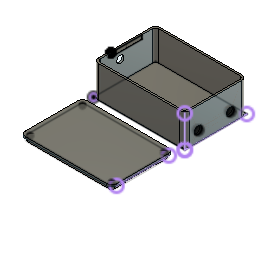
esp12_triac v6 (Autodesk Fusion 360 design; units mm, degrees)
Autodesk Fusion 360 part; units mm, degrees
sketch "Base" plane through (0, 0, 0) normal (0, 1, 0) x (1, 0, 0) in component "Case"
  line L0 (0, 0) -> (75, 0)
  line L1 (75, 0) -> (75, 51)
  line L2 (75, 51) -> (0, 51)
  line L3 (0, 51) -> (0, 0)
  dimension "d6" = 75
  dimension "d7" = 51
  constraint horizontal L0
  constraint vertical L1
  constraint horizontal L2
  constraint vertical L3
  constraint coincident L0.start L3.end
  measures "d6" distance of L0.start L0.end
  measures "d7" distance of L0.start L2.end
extrude "Extrude1" add sketch "Base" along normal blind 26 makes body 1 in component "Case"
fillet "Fillet1" radius 4 4 edges at (75, 13, 0) (0, 13, 0) (75, 13, -51) (0, 13, -51) on bodies 1 in component "Case"
shell "Shell1" thickness 1.5 removed faces 1 at (48.6667, 26, -17) on bodies 1 in component "Case"
sketch "Knob" plane through (1.5, 0, 0) normal (1, 0, 0) x (0, 0, -1) in component "Case"
  line L0 (47, 1.5) -> (47, 26)
  line L1 (47, 26) -> (4, 26)
  line L2 (4, 26) -> (4, 1.5)
  line L3 (4, 1.5) -> (47, 1.5)
  line L4 (12.75, 26) -> (38.25, 26)
  line L5 (38.25, 26) -> (38.25, 23)
  line L6 (38.25, 23) -> (12.75, 23)
  line L7 (12.75, 23) -> (12.75, 26)
  line L8 (25.5, 26) -> (25.5, 23) construction
  dimension "d12" = 25.5
  dimension "d13" = 3
  constraint horizontal L4
  constraint vertical L5
  constraint horizontal L6
  constraint vertical L7
  constraint coincident L1 L4.start
  constraint midpoint L1 L8.start
  constraint midpoint L6 L8.end
  constraint vertical L8
  measures "d12" distance of L5.end L6.end
  measures "d13" distance of L4.end L5.end
extrude "Extrude2" add sketch "Knob" along normal blind 6 draft -45 contours L1 L4 L5 L6 L7 bodies 1 in component "Case"
ref_plane "WorkPlane2" through (37.5, 13, -25.5) normal (-1, 0, 0) x (0, 0, 1) in component "Case"
mirror "Mirror1" about plane through (37.5, 13, -25.5) normal (-1, 0, 0) of "Extrude2" in component "Case"
sketch "Top" plane through (0, 26, 0) normal (0, 1, 0) x (-1, 0, 0) in component "Top Cover"
  line L0 (-75, -4) -> (-75, -47)
  arc A0 (-75, -47) -> (-71, -51) centre (-71, -47) ccw
  line L1 (-71, -51) -> (-4, -51)
  arc A1 (-4, -51) -> (0, -47) centre (-4, -47) ccw
  line L2 (0, -47) -> (0, -4)
  arc A2 (0, -4) -> (-4, 0) centre (-4, -4) ccw
  line L3 (-4, 0) -> (-71, 0)
  arc A3 (-71, 0) -> (-75, -4) centre (-71, -4) ccw
  line L4 (-73.5, -12.75) -> (-73.5, -4)
  arc A4 (-71, -1.5) -> (-73.5, -4) centre (-71, -4) ccw
  line L5 (-71, -1.5) -> (-4, -1.5)
  arc A5 (-1.5, -4) -> (-4, -1.5) centre (-4, -4) ccw
  line L6 (-1.5, -4) -> (-1.5, -12.75)
  line L7 (-1.5, -12.75) -> (-1.5, -38.25)
  line L8 (-1.5, -38.25) -> (-1.5, -47)
  arc A6 (-4, -49.5) -> (-1.5, -47) centre (-4, -47) ccw
  line L9 (-4, -49.5) -> (-71, -49.5)
  arc A7 (-73.5, -47) -> (-71, -49.5) centre (-71, -47) ccw
  line L10 (-73.5, -47) -> (-73.5, -38.25)
  line L11 (-73.5, -38.25) -> (-73.5, -12.75)
extrude "Extrude1'" add sketch "Top" along normal blind 1.5 separate body contours L0 A0 L1 A1 L2 A2 L3 A3 | L4 A4 L5 A5 L6 L7 L8 A6 L9 A7 L10 L11 makes body 2 in component "Top Cover"
sketch "Lip" plane through (0, 26, 0) normal (0, -1, 0) x (1, 0, 0) in component "Top Cover"
  arc A0 (75, -4) -> (71, 0) centre (71, -4) ccw
  line L0 (71, 0) -> (4, 0)
  arc A1 (4, 0) -> (0, -4) centre (4, -4) ccw
  line L1 (0, -4) -> (0, -47)
  arc A2 (0, -47) -> (4, -51) centre (4, -47) ccw
  line L2 (4, -51) -> (71, -51)
  arc A3 (71, -51) -> (75, -47) centre (71, -47) ccw
  line L3 (75, -47) -> (75, -4)
  line L4 (73.3, -47) -> (73.3, -4)
  arc A4 (73.3, -4) -> (71, -1.7) centre (71, -4) ccw
  line L5 (71, -1.7) -> (4, -1.7)
  arc A5 (4, -1.7) -> (1.7, -4) centre (4, -4) ccw
  line L6 (1.7, -4) -> (1.7, -47)
  arc A6 (1.7, -47) -> (4, -49.3) centre (4, -47) ccw
  line L7 (4, -49.3) -> (71, -49.3)
  arc A7 (71, -49.3) -> (73.3, -47) centre (71, -47) ccw
  line L8 (75, -4) -> (75, -47)
  dimension "d19" = 1.7
  dimension "d31" = 1.7
  measures "d31" distance of L4 L8
extrude "Extrude2'" add sketch "Lip" along normal blind 3 contours L4 A4 L5 A5 L6 A6 L7 A7 bodies 2 in component "Top Cover"
extrude "Extrude3" cut sketch "Knob" along normal blind 3 draft -45 from surface at 0.2 contours L1 L4 L5 L6 L7 bodies 2 in component "Top Cover"
ref_plane "WorkPlane2" through (37.5, 0, 0) normal (1, 0, 0) x (0, 1, 0) in component "Top Cover"
mirror "Mirror1'" about plane through (37.5, 0, 0) normal (1, 0, 0) of "Extrude3" in component "Top Cover"
shell "Shell1'" thickness 1.5 removed faces 1 at (49.4333, 23, -29.75) on bodies 2 in component "Top Cover"
chamfer "Chamfer1" distance 0.6 angle 45 2 edges at (1.7, 23, -25.5) (73.3, 23, -25.5) on bodies 2 in component "Top Cover"
sketch "Esquisse1" plane through (75, 0, 0) normal (1, 0, 0) x (0, 0, -1)
  line L0 (47, 26) -> (4, 26)
  line L1 (4, 26) -> (4, 0)
  line L2 (4, 0) -> (47, 0)
  line L3 (47, 0) -> (47, 26)
  circle A0 centre (11, 8.5) radius 3
  line L4 (0, 26) -> (0, 0)
  line L5 (0, 0) -> (51, 0)
  circle A1 centre (37.5, 8.5) radius 3
  dimension "d37" = 6
  dimension "d38" = 11
  dimension "d39" = 8.5
  dimension "d40" = 6
  dimension "d42" = 8.5
  dimension "d43" = 26.5
  measures "d37" diameter of A0
  measures "d38" distance of A0.centre L4
  measures "d39" distance of A0.centre L5
  measures "d40" diameter of A1
  measures "d42" distance of L5 A1.centre
  measures "d43" distance of A0.centre A1.centre
extrude "Extrusion4" cut sketch "Esquisse1" against normal blind 1.6 contours A0 | A1 bodies 1 in component "Case"
sketch "Esquisse2" plane through (0, 0, 0) normal (-1, 0, 0) x (0, 0, 1)
  line L0 (-47, 26) -> (-47, 0)
  line L1 (-47, 0) -> (-4, 0)
  line L2 (-4, 0) -> (-4, 26)
  line L3 (-4, 26) -> (-47, 26)
  circle A0 centre (-20.5, 17.5) radius 3
  line L4 (-51, 0) -> (0, 0)
  dimension "d49" = 6
  dimension "d50" = 20.5
  dimension "d53" = 17.5
  measures "d49" diameter of A0
  measures "d50" horizontal distance of A0.centre L4.end
  measures "d53" distance of A0.centre L4
extrude "Extrusion5" cut sketch "Esquisse2" against normal blind 1.6 contours A0 bodies 1 in component "Case"
component "Enclosure" placed x (1, 0, 0) y (0, 1, 0) z (0, 0, 1) at (0, 0, 0)
component "Case" placed x (1, 0, 0) y (0, 1, 0) z (0, 0, 1) at (0, 0, 0) in component "Enclosure"
component "Top Cover" placed x (1, 0, 0) y (0, 1, 0) z (0, 0, 1) at (0, 0, 0) in component "Enclosure"
equation "Width = Width_internal + ( 2 * shell )"
equation "length = Length_internal + ( 2 * shell )"
equation "heigth = Height_internal + ( 2 * shell )"
equation "shell = 1.5 mm"
equation "gap = 0.2 mm"
equation "d6 = length"
equation "d7 = Width"
equation "d8 = heigth"
equation "d11 = shell"
equation "d12 = Width / 2"
equation "d13 = shell * 2"
equation "d17 = shell"
equation "d19 = shell + gap"
equation "d20 = shell * 2"
equation "d23 = shell * 2"
equation "d26 = shell"
equation "d31 = shell + gap"
equation "d33 = length / 2"
equation "Width_internal = 48 mm"
equation "Length_internal = 72 mm"
equation "Height_internal = 23 mm"
equation "d37 = wire_hole"
equation "d38 = 9.5 mm + shell"
equation "d39 = 7 mm + shell"
equation "d40 = wire_hole"
equation "wire_hole = 6 mm"
equation "d42 = d39"
equation "d46 = -( shell + 0.1 mm )"
equation "button_hole = 6 mm"
equation "d49 = button_hole"
equation "d50 = 19 mm + shell"
equation "d51 = -( shell + 0.1 mm )"
equation "d53 = Height_internal + shell - button_hole / 2 - 4 mm"
